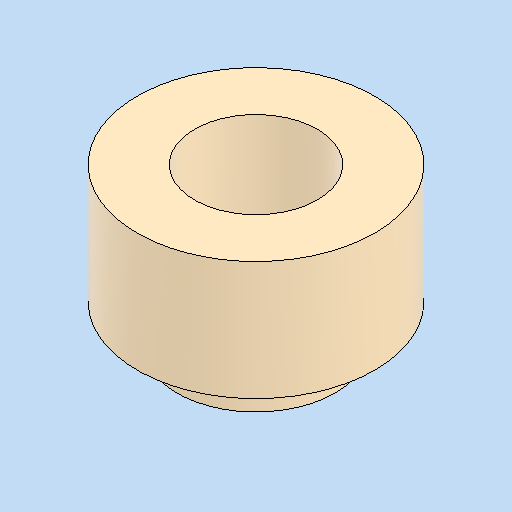
# Autodesk Inventor part: Ceramic Bushing M3 V1
Saved by Autodesk Inventor 2025 (Build 290162000, 162)
## iProperties
Created: 2019-11-08
Part Number: Ceramic Bushing M3 V1
Material: Silicon Nitride
Document SubType Name: Modeling
Designer: kuzmin
Density: 3.18 g/cm^3
Appearance: Smooth - Off-White
Mass: 0.449437 g
Surface Area: 2.51626 cm^2
Volume: 0.141332 cm^3
Author: kuzmin
Autodesk Inventor part; units mm, degrees
ref_plane "YZ Plane" through (0, 0, 0) normal (1, 0, 0) x (0, 1, 0)
ref_plane "XZ Plane" through (0, 0, 0) normal (0, 1, 0) x (-1, 0, 0)
ref_plane "XY Plane" through (0, 0, 0) normal (0, 0, 1) x (1, 0, 0)
sketch "Sketch1" plane through (0, 0, 0) normal (0, 0, 1) x (1, 0, 0)
  line L0 (2, 0) -> (2, 1)
  line L1 (2, 1) -> (3, 1)
  line L2 (3, 1) -> (3, 4)
  line L3 (3, 4) -> (1.55, 4)
  line L4 (1.55, 4) -> (1.55, 0)
  line L5 (0, 0) -> (0, 8.8913)
  line L6 (1.55, 0) -> (2, 0)
  dimension "d0" = 4
  dimension "d1" = 1
  dimension "d2" = 3
  dimension "d3" = 3.1
  dimension "d4" = 6
  constraints: 14 end point, 3 perpendicular, 1 horizontal, 1 vertical
  measures "d0" diameter of L0 L5
  measures "d1" distance of L0.start L0.end
  measures "d2" distance of L1.end L2.end
  measures "d3" diameter of L4 L5
  measures "d4" diameter of L2 L5
revolve "Revolution1" add sketch "Sketch1" angle 360 about axis through (0, 0, 0) along (0, 1, 0)
equation "\"d0\" = od_b"
equation "\"d1\" = t2"
equation "\"d2\" = t1"
equation "\"d3\" = id"
equation "\"d4\" = od_a"
equation "\"od_a\" = 6"
equation "\"od_b\" = 4"
equation "\"t1\" = 3"
equation "\"t2\" = 1"
equation "\"id\" = 3.1"
body "Solid1"
